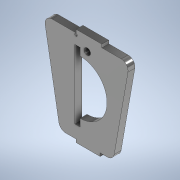
# Autodesk Inventor part: Part41
Saved by Autodesk Inventor 2021 (Build 250183000, 183)
## iProperties
Created: 2020-11-06
Part Number: Part41
Material: Liga de Nickel-Copper 400
Document SubType Name: Modeling
Designer: pedro
Density: 8.83 g/cm^3
Appearance: Cromado - Preto polido
Author: pedro
Autodesk Inventor part; units mm, degrees
ref_plane "YZ Plane" through (0, 0, 0) normal (1, 0, 0) x (0, 1, 0)
ref_plane "XZ Plane" through (0, 0, 0) normal (0, 1, 0) x (-1, 0, 0)
ref_plane "XY Plane" through (0, 0, 0) normal (0, 0, 1) x (1, 0, 0)
sketch "Sketch1" plane through (0, 0, 0) normal (0, 0, 1) x (1, 0, 0)
  line L0 (-4.5, -0.0453) -> (4.5, -0.0453)
  line L1 (4.5, -0.0453) -> (4.5, 0.8547)
  line L2 (4.5, 0.8547) -> (4.6, 0.8547)
  line L3 (6.5696, 2.5074) -> (10.5639, 25.1601)
  arc A0 (4.6, 0.8547) -> (6.5696, 2.5074) centre (4.6, 2.8547) ccw
  line L4 (-4.5, -0.0453) -> (-4.5, 0.8547)
  line L5 (-4.5, 0.8547) -> (-7.5, 0.8547)
  line L6 (-9.4696, 2.5074) -> (-13.4639, 25.1601)
  arc A1 (-9.4696, 2.5074) -> (-7.5, 0.8547) centre (-7.5, 2.8547) ccw
  line L7 (10.9778, 27.5074) -> (-13.8778, 27.5074) construction
  line L8 (-4.5, -0.7454) -> (-4.5, 29.497) construction
  line L9 (-4.5, 31.0971) -> (4.5, 31.0971) construction
  line L10 (4.5, 31.0971) -> (4.5, 0.8547) construction
  line L11 (8.5943, 27.5074) -> (4.5, 27.5074)
  line L12 (-11.4943, 27.5074) -> (-4.5, 27.5074)
  line L13 (4.5, 27.5074) -> (4.5, 28.4074)
  line L14 (-4.5, 28.4074) -> (-4.5, 27.5074)
  line L15 (-4.5, 28.4074) -> (4.5, 28.4074)
  arc A2 (10.5639, 25.1601) -> (8.5943, 27.5074) centre (8.5943, 25.5074) ccw
  arc A3 (-11.4943, 27.5074) -> (-13.4639, 25.1601) centre (-11.4943, 25.5074) ccw
  arc A4 (-3.3267, 6.6293) -> (-3.3267, 22.2828) centre (-3.3267, 14.456) ccw
  line L16 (-3.3267, 24.456) -> (-3.3267, 14.456)
  line L17 (-3.3267, 14.456) -> (-3.3267, 4.456)
  line L18 (-3.3267, 4.456) -> (-4.5, 4.456)
  line L19 (-3.3267, 24.456) -> (-4.5, 24.456)
  line L20 (-4.5, 4.4448) -> (-4.5, 24.4448)
  circle A5 centre (7.1554, 22.5114) radius 0.4516
  circle A6 centre (-1.2395, 24.4257) radius 0.9502
  circle A7 centre (-4.5, 27.0227) radius 0.3751
  point P0 (0, 0)
  dimension "d1" = 2
  dimension "d2" = 100
  dimension "d3" = 25
  dimension "d4" = 0.1
  dimension "d5" = 2
  dimension "d6" = 3
  dimension "d7" = 4.5
  dimension "d8" = 4.5
  dimension "d9" = 100
  dimension "d10" = 25
  dimension "d11" = 0.9
  dimension "d12" = 0.9
  dimension "d13" = 2
  dimension "d16" = 10
  dimension "d17" = 10
  constraints: 42 end point, 13 point on line, 10 point on circle, 9 perpendicular, 8 centre point, 8 tangent, 3 vertical, 1 collinear, 1 equal radius, 1 horizontal
  measures "d1" radius of A0
  measures "d2" angle of L2 L3
  measures "d3" vertical distance of L3.start L7.start
  measures "d4" distance of L1.end L2.end
  measures "d5" radius of A1
  measures "d6" distance of L5.start L5.end
  measures "d7" horizontal distance of L0.start point (0, 0)
  measures "d8" horizontal distance of L0.end point (0, 0)
  measures "d9" angle of L5 L6
  measures "d10" vertical distance of L6.start L7.end
  measures "d11" distance of L0.end L1.end
  measures "d12" distance of L14.start L12.end
  measures "d13" radius of A2
  measures "d16" distance of L16.end L17.end
  measures "d17" distance of L16.start L16.end
extrude "Extrusion1" add sketch "Sketch1" along normal mid plane 2 contours L4 L5 A1 L6 A3 L12 L14 L15 L13 L11 A2 L3 A0 L2 L1 L0 | L17 L16 A4 | A5 | A6 | A7
extrude "Extrusion2" cut sketch "Sketch1" against normal through all contours L17 L16 A4
extrude "Extrusion3" cut sketch "Sketch1" along normal through all both and the other way through all contours L17 L16 A4
extrude "Extrusion6" cut sketch "Sketch1" against normal through all both and the other way through all contours A6
extrude "Extrusion7" cut sketch "Sketch1" against normal through all both and the other way through all contours A7
sketch "Esboço2" plane through (4.5, -0.0453, 1) normal (1, 0, 0) x (0, 0, -1)
  line L0 (0, 0.9) -> (2, 0.9) projected
  line L1 (0, 0.9) -> (2, 0.9)
  line L2 (2, 0) -> (0, 0) projected
  line L3 (2, 0.9) -> (2, 0)
  line L4 (2, 0) -> (0, 0)
  line L5 (0, 0) -> (0, 0.9) projected
  line L6 (0, 0) -> (0, 0.9)
  point P0 (1, 0.0453)
  constraints: 8 end point, 2 perpendicular, 1 collinear, 1 horizontal
extrude "Extrusão8" cut sketch "Esboço2" against normal blind 2
sketch "Esboço3" plane through (4.5, 27.5074, 1) normal (1, 0, 0) x (0, 0, -1)
  line L0 (2, 0.9) -> (0, 0.9) projected
  line L1 (0, 0.9) -> (2, 0.9)
  line L2 (2, 0) -> (0, 0) projected
  line L3 (2, 0.9) -> (2, 0)
  line L4 (2, 0) -> (0, 0)
  line L5 (0, 0.9) -> (0, 0) projected
  line L6 (0, 0) -> (0, 0.9)
  point P0 (1, -27.5074)
  constraints: 8 end point, 3 perpendicular, 1 collinear
extrude "Extrusão9" cut sketch "Esboço3" against normal blind 1.5
sketch "Esboço4" plane through (0, 0, 1) normal (0, 0, 1) x (1, 0, 0)
  line L0 (-3.3267, 22.2828) -> (-3.3267, 6.6293) projected
  line L1 (-3.3267, 22.2828) -> (-3.3267, 24.456)
  line L2 (-3.3267, 24.456) -> (-4.8267, 24.456)
  line L3 (-4.8267, 24.456) -> (-4.8267, 4.456)
  line L4 (-4.8267, 4.456) -> (-3.3267, 4.456)
  line L5 (-3.3267, 4.456) -> (-3.3267, 6.6293)
  arc A0 (-3.3267, 6.6293) -> (-3.3267, 22.2828) centre (-3.3267, 14.456) ccw projected
  point P0 (0, 0)
  dimension "d36" = 20
  dimension "d37" = 1.5
  dimension "d38" = 10
  constraints: 10 end point, 4 perpendicular, 1 point on line, 1 vertical
  measures "d36" distance between parallel lines of L2 L4
  measures "d37" distance between parallel lines of L0 L3
  measures "d38" distance from line of A0.centre L2
extrude "Extrusão10" cut sketch "Esboço4" against normal blind 10 contours L0 L5 L4 L3 L2 L1
body "Solid1"
